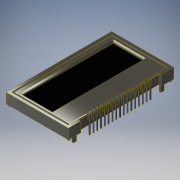
# Autodesk Inventor part: NHD-C12832A1Z_LCD
Saved by Autodesk Inventor 2016 (Build 200138000, 138)
## iProperties
Created: 2016-09-06
Part Number: NHD-C12832A1Z_LCD
Material: Generic
Document SubType Name: Modeling
Designer: jfixelle
Density: 1 g/cm^3
Appearance: Silver
Author: jfixelle
Autodesk Inventor part; units mm, degrees
ref_plane "YZ Plane" through (0, 0, 0) normal (1, 0, 0) x (0, 1, 0)
ref_plane "XZ Plane" through (0, 0, 0) normal (0, 1, 0) x (-1, 0, 0)
ref_plane "XY Plane" through (0, 0, 0) normal (0, 0, 1) x (1, 0, 0)
sketch "Sketch1" plane through (0, 0, 0) normal (0, 1, 0) x (-1, 0, 0)
  line L0 (11.25, 19.8) -> (-11.25, 19.8)
  line L1 (-11.25, 19.8) -> (-11.25, -19.8)
  line L2 (-11.25, -19.8) -> (11.25, -19.8)
  line L3 (11.25, -19.8) -> (11.25, 19.8)
  point P0 (0, 0)
  dimension "d0" = 39.6
  dimension "d1" = 22.5
  dimension "d2" = 11.25
  dimension "d3" = 19.8
  constraints: 8 end point, 2 parallel, 1 horizontal, 1 perpendicular
  measures "d0" distance of L2.end L0.start
  measures "d1" distance of L1.end L2.end
  measures "d2" distance from line of point (0, 0) L3
  measures "d3" distance from line of point (0, 0) L2
extrude "Extrusion1" add sketch "Sketch1" along normal blind 4
fillet "Fillet1" radius 0.5 4 edges at (0, 4, 19.8) (11.25, 4, 0) (-11.25, 4, 0) (0, 4, -19.8)
sketch "Sketch2" plane through (0, 0, 0) normal (0, -1, 0) x (1, 0, 0)
  line L0 (-12.3, 20.85) -> (12.3, 20.85)
  line L1 (12.3, -20.85) -> (-12.3, -20.85)
  line L2 (-12.3, -20.85) -> (-12.3, 20.85)
  line L3 (12.3, 15.99) -> (11.25, 15.99)
  line L4 (11.25, 19.8) -> (11.25, -19.8) projected
  line L5 (12.3, -15.99) -> (11.25, -15.99)
  line L6 (11.25, -15.99) -> (11.25, 15.99)
  line L7 (12.3, 20.85) -> (12.3, 15.99)
  line L8 (12.3, -15.99) -> (12.3, -20.85)
  line L9 (-11.25, 19.8) -> (11.25, 19.8) projected
  line L10 (-11.25, 19.8) -> (11.25, 19.8)
  line L11 (11.25, 19.8) -> (11.25, -19.8)
  line L12 (11.25, -19.8) -> (-11.25, -19.8)
  line L13 (-11.25, -19.8) -> (-11.25, 19.8)
  point P0 (0, 0)
  dimension "d7" = 24.6
  dimension "d8" = 41.7
  dimension "d9" = 20.85
  dimension "d10" = 12.3
  dimension "d11" = 31.98
  dimension "d12" = 15.99
  constraints: 24 end point, 6 parallel, 3 horizontal, 3 perpendicular, 2 point on line, 1 collinear
  measures "d7" distance of L0.start L0.end
  measures "d8" distance of L1.end L0.start
  measures "d9" distance from line of point (0, 0) L1
  measures "d10" distance from line of point (0, 0) L2
  measures "d11" distance between parallel lines of L5 L3
  measures "d12" distance from line of point (0, 0) L3
extrude "Extrusion2" add sketch "Sketch2" against normal blind 4 contours L0 L7 L3 L4 L9 L13 L12 L5 L8 L1 L2
sketch "Sketch3" plane through (0, 4, 0) normal (0, 1, 0) x (1, 0, 0)
  line L0 (-8.85, -18) -> (3.15, -18)
  line L1 (3.15, -18) -> (3.15, 18)
  line L2 (3.15, 18) -> (-8.85, 18)
  line L3 (-8.85, 18) -> (-8.85, -18)
  line L4 (-10.75, -19.3) -> (-10.75, 19.3) projected
  point P0 (0, 0)
  dimension "d15" = 12
  dimension "d16" = 36
  dimension "d17" = 18
  dimension "d18" = 1.9
  constraints: 8 end point, 2 parallel, 1 horizontal, 1 perpendicular
  measures "d15" distance of L0.start L0.end
  measures "d16" distance of L2.end L0.start
  measures "d17" distance from line of point (0, 0) L0
  measures "d18" distance between parallel lines of L4 L3
extrude "Extrusion3" cut sketch "Sketch3" against normal blind 1
chamfer "Chamfer1" distance 0.5 angle 45 4 edges at (-2.85, 4, 18) (3.15, 4, 0) (-8.85, 4, 0) (-2.85, 4, -18)
sketch "Sketch5" plane through (0, 4, 0) normal (0, 1, 0) x (1, 0, 0)
  circle A0 centre (11.7, 12.15) radius 0.25
  line L0 (12.3, 20.85) -> (-12.3, 20.85) projected
  line L1 (12.3, 15.99) -> (12.3, 20.85) projected
  point P0 (0, 0)
  dimension "d26" = 0.5
  dimension "d27" = 8.7
  dimension "d28" = 0.6
  constraints: 1 centre point
  measures "d26" diameter of A0
  measures "d27" distance from line of L0 A0.centre
  measures "d28" distance from line of A0.centre L1
extrude "Extrusion4" add sketch "Sketch5" against normal blind 7
sketch "Sketch6" plane through (11.7, 4, -12.15) normal (0, 1, 0) x (1, 0, 0)
  line L0 (0.3017, 0.3392) -> (-1.1311, 0.3392)
  line L1 (-1.1311, 0.3392) -> (-1.1311, -0.3262)
  line L2 (-1.1311, -0.3262) -> (0.3017, -0.3262)
  line L3 (0.3017, -0.3262) -> (0.3017, 0.3392)
  point P0 (-11.7, -12.15)
  constraints: 8 end point, 2 parallel, 1 horizontal, 1 perpendicular
extrude "Extrusion5" add sketch "Sketch6" against normal blind 2
pattern_linear "Rectangular Pattern1" count 17 spacing 1.5 along (0, 0, 1) of "Extrusion4", "Extrusion5"
sketch "Sketch7" plane through (0, 0, 0) normal (0, -1, 0) x (1, 0, 0)
  line L0 (11.375, 17.9) -> (10.675, 17.9)
  line L1 (10.675, 17.9) -> (10.675, 16.7)
  line L2 (10.675, 16.7) -> (11.375, 16.7)
  line L3 (11.375, 16.7) -> (11.375, 17.9)
  line L4 (12.3, 15.99) -> (12.3, 20.85) projected
  point P0 (0, 0)
  dimension "d36" = 1.2
  dimension "d37" = 0.7
  dimension "d38" = 16.7
  dimension "d39" = 0.925
  constraints: 8 end point, 2 parallel, 1 horizontal, 1 perpendicular
  measures "d36" distance of L2.end L0.start
  measures "d37" distance of L1.end L2.end
  measures "d38" distance from line of point (0, 0) L2
  measures "d39" distance between parallel lines of L4 L3
extrude "Extrusion6" add sketch "Sketch7" along normal blind 3
mirror "Mirror1" about plane through (0, 0, 0) normal (0, 0, 1) of "Extrusion6"
sketch "Sketch8" plane through (0, 0, 0) normal (0, -1, 0) x (1, 0, 0)
  circle A0 centre (11.7, 20.1) radius 0.4
  circle A1 centre (11.7, -20.1) radius 0.4
  circle A2 centre (-11.7, -20.1) radius 0.4
  circle A3 centre (-11.7, 20.1) radius 0.4
  line L0 (-12.3, 20.85) -> (-12.3, -20.85) projected
  line L1 (12.3, -20.85) -> (12.3, -15.99) projected
  point P0 (0, 0)
  dimension "d42" = 0.8
  dimension "d43" = 0.8
  dimension "d44" = 0.8
  dimension "d45" = 0.8
  dimension "d46" = 40.2
  dimension "d47" = 20.1
  dimension "d48" = 40.2
  dimension "d49" = 20.1
  dimension "d50" = 0
  dimension "d51" = 0
  dimension "d52" = 0.6
  dimension "d53" = 0.6
  constraints: 4 centre point
  measures "d42" diameter of A3
  measures "d43" diameter of A2
  measures "d44" diameter of A1
  measures "d45" diameter of A0
  measures "d46" distance of A2.centre A3.centre
  measures "d47" vertical distance of point (0, 0) A2.centre
  measures "d48" distance of A1.centre A0.centre
  measures "d49" vertical distance of point (0, 0) A1.centre
  measures "d50" horizontal distance of A1.centre A0.centre
  measures "d51" horizontal distance of A3.centre A2.centre
  measures "d52" distance from line of L0 A2.centre
  measures "d53" distance from line of A1.centre L1
extrude "Extrusion7" add sketch "Sketch8" along normal blind 0.9
fillet "Fillet2" radius 0.3 4 edges at (-12.1, -0.9, 20.1) (-12.1, -0.9, -20.1) (11.3, -0.9, -20.1) (11.3, -0.9, 20.1)
body "Solid1"
